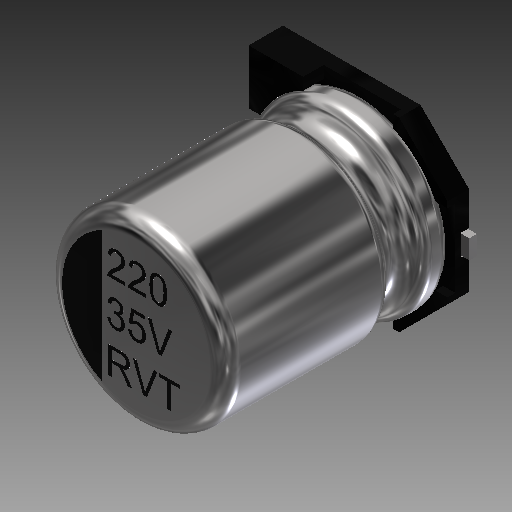
# Autodesk Inventor part: CAPSMD220-35
Saved by Autodesk Inventor 2018 (Build 220112000, 112)
## iProperties
Created: 2017-08-07
Part Number: CAPSMD220-35
Material: Generic
Document SubType Name: Modeling
Designer: joseph.strelchuk
Manufacturer: Standard
Standards Organization: Custom
Density: 1 g/cm^3
Appearance: Semi-Polished
Author: joseph.strelchuk
Autodesk Inventor part; units mm, degrees
ref_plane "YZ Plane" through (0, 0, 0) normal (1, 0, 0) x (0, 1, 0)
ref_plane "XZ Plane" through (0, 0, 0) normal (0, 1, 0) x (-1, 0, 0)
sketch "Sketch11" plane through (0, 0, 0) normal (0, 0, 1) x (1, 0, 0)
  line L0 (-4.15, -4.15) -> (4.15, -4.15)
  line L1 (4.15, -4.15) -> (4.15, 4.15)
  line L2 (4.15, 4.15) -> (-4.15, 4.15)
  line L3 (-4.15, 4.15) -> (-4.15, -4.15)
  line L4 (-4.15, -4.15) -> (4.15, 4.15) construction
  line L5 (4.15, -4.15) -> (-4.15, 4.15) construction
  point P0 (0, 0)
  dimension "d50" = 8.3
  dimension "d51" = 8.3
  constraints: 12 end point, 2 midpoint, 2 parallel, 1 horizontal, 1 perpendicular
  measures "d50" distance of L2.end L1.end
  measures "d51" distance of L1.end L0.end
extrude "Extrusion9" add sketch "Sketch11" along normal blind 1.53
chamfer "Chamfer1" distance 2.16 distance2 2.16 1 edges at (4.15, -4.15, 0.765) measured on face at (-1.3833, -4.15, 0.51)
chamfer "Chamfer2" distance 2.16 distance2 2.16 1 edges at (4.15, 4.15, 0.765) measured on face at (4.15, 0.0567, 0.51)
sketch "Sketch12" plane through (0, 0, 1.53) normal (0, 0, 1) x (1, 0, 0)
  line L0 (4.15, -1.99) -> (1.99, -4.15) construction
  line L1 (1.99, -4.15) -> (-4.15, -4.15) construction
  line L2 (-4.15, -4.15) -> (-4.15, 4.15) construction
  line L3 (-4.15, 4.15) -> (1.99, 4.15) construction
  line L4 (1.99, 4.15) -> (4.15, 1.99) construction
  line L5 (4.15, 1.99) -> (4.15, -1.99) construction
  line L6 (-4.15, 0) -> (4.15, 0) construction
  line L7 (0, 4.15) -> (0, -4.15) construction
  line L8 (-4.15, 1.72) -> (-4.15, -1.72)
  line L9 (-4.15, 4.15) -> (-4.15, -4.15) projected
  line L10 (-1.72, 4.15) -> (1.72, 4.15)
  line L11 (4.15, 1.72) -> (4.15, -1.72)
  line L12 (-1.72, -4.15) -> (1.72, -4.15)
  line L13 (4.15, -1.99) -> (4.15, 1.99) projected
  line L14 (-4.15, -1.72) -> (-3.6113, -1.72)
  line L15 (-4.15, 1.72) -> (-3.6113, 1.72)
  line L16 (-1.72, 4.15) -> (-1.72, 3.6113)
  line L17 (1.72, 4.15) -> (1.72, 3.6113)
  line L18 (4.15, 1.72) -> (3.6113, 1.72)
  line L19 (4.15, -1.72) -> (3.6113, -1.72)
  line L20 (1.72, -4.15) -> (1.72, -3.6113)
  line L21 (-1.72, -4.15) -> (-1.72, -3.6113)
  arc A0 (-3.6113, -1.72) -> (-1.72, -3.6113) centre (0, 0) ccw
  arc A1 (-1.72, 3.6113) -> (-3.6113, 1.72) centre (0, 0) ccw
  arc A2 (1.72, -3.6113) -> (3.6113, -1.72) centre (0, 0) ccw
  arc A3 (3.6113, 1.72) -> (1.72, 3.6113) centre (0, 0) ccw
  dimension "d64" = 3.44
  dimension "d65" = 3.44
  dimension "d66" = 3.44
  dimension "d67" = 3.44
  dimension "d68" = 4
  dimension "d69" = 4
  dimension "d70" = 4
  dimension "d71" = 4
  constraints: 28 end point, 10 midpoint, 8 point on circle, 4 centre point, 4 horizontal, 4 perpendicular, 3 vertical, 2 parallel, 2 point on line, 1 coincident
  measures "d64" distance of L8.start L8.end
  measures "d65" distance of L10.start L10.end
  measures "d66" distance of L11.start L11.end
  measures "d67" distance of L12.start L12.end
  measures "d68" radius of A3
  measures "d69" radius of A1
  measures "d70" radius of A2
  measures "d71" radius of A0
extrude "Extrusion10" cut sketch "Sketch12" against normal blind 0.92
sketch "Sketch13" plane through (0, 0, 1.53) normal (0, 0, 1) x (1, 0, 0)
  line L0 (3.6113, 1.72) -> (4.15, 1.72) projected
  line L1 (4.15, 1.72) -> (4.15, 1.99) projected
  line L2 (1.99, 4.15) -> (4.15, 1.99) projected
  line L3 (1.99, 4.15) -> (1.72, 4.15) projected
  line L4 (1.72, 4.15) -> (1.72, 3.6113) projected
  arc A0 (3.6113, 1.72) -> (1.72, 3.6113) centre (0, 0) ccw projected
  line L5 (4.15, -1.72) -> (3.6113, -1.72) projected
  arc A1 (1.72, -3.6113) -> (3.6113, -1.72) centre (0, 0) ccw projected
  line L6 (1.72, -3.6113) -> (1.72, -4.15) projected
  line L7 (1.72, -4.15) -> (1.99, -4.15) projected
  line L8 (4.15, -1.99) -> (1.99, -4.15) projected
  line L9 (4.15, -1.99) -> (4.15, -1.72) projected
extrude "Extrusion11" cut sketch "Sketch13" against normal blind 0.57
ref_plane "Work Plane1" through (4.15, 0, 0) normal (0, -1, 0) x (0, 0, 1)
sketch "Sketch14" plane through (4.15, 0, 0) normal (0, -1, 0) x (0, 0, 1)
  line L0 (0.61, 2.43) -> (0.61, 5.87) projected
  line L1 (0, 8.3) -> (0, 2.16) projected
  line L2 (0.61, 4.15) -> (10.72, 4.15)
  line L3 (0.61, 4.15) -> (10.7, 4.15)
  line L4 (10.7, 4.15) -> (10.7, 0.85)
  line L5 (0.61, 0.65) -> (0.61, 4.15)
  arc A0 (10, 0.15) -> (10.7, 0.85) centre (10, 0.85) ccw
  line L6 (0.61, 4.15) -> (2.61, 4.15) construction
  line L7 (2.61, 4.15) -> (2.61, 0.15) construction
  arc A1 (3.2974, 0.45) -> (1.9226, 0.45) centre (2.61, 0.15) ccw
  line L8 (10, 0.15) -> (3.7556, 0.15)
  line L9 (1.4644, 0.15) -> (1.11, 0.15)
  arc A2 (3.2974, 0.45) -> (3.7556, 0.15) centre (3.7556, 0.65) ccw
  arc A3 (1.4644, 0.15) -> (1.9226, 0.45) centre (1.4644, 0.65) ccw
  arc A4 (0.61, 0.65) -> (1.11, 0.15) centre (1.11, 0.65) ccw
  point P0 (0, 4.15)
  point P1 (10.7, 0.15)
  point P2 (3.36, 0.15)
  point P3 (1.86, 0.15)
  point P4 (0.63, 2.1134)
  point P5 (0.63, 6.892)
  dimension "d74" = 10.72
  dimension "d75" = 4
  dimension "d76" = 0.7
  dimension "d77" = 2
  dimension "d78" = 1.5
  dimension "d79" = 0.5
  dimension "d80" = 0.3544
  dimension "d81" = 4
  dimension "d82" = 6.2444
  constraints: 16 end point, 12 point on circle, 9 tangent, 5 centre point, 4 point on line, 3 parallel, 3 perpendicular, 2 equal radius, 2 horizontal, 1 coincident, 2 other
  measures "d74" distance from line of L1 L2.end
  measures "d75" distance of L3.end point (10.7, 0.15)
  measures "d76" radius of A0
  measures "d77" distance of L2.start L6.end
  measures "d78" diameter of A1
  measures "d79" radius of A2
  measures "d80" distance of L9.start L9.end
  measures "d81" distance of L6.end L7.end
  measures "d82" distance of L8.start L8.end
revolve "Revolution1" add sketch "Sketch14" angle 360 about axis through (0, 0, 0.61) along (0, 0, 1)
sketch "Sketch15" plane through (0, 0, 0) normal (0, 0, -1) x (-1, 0, 0)
  line L0 (4.5, 0.425) -> (1.12, 0.425) construction
  line L1 (1.12, 0.425) -> (1.12, -0.425) construction
  line L2 (1.12, -0.425) -> (4.5, -0.425) construction
  line L3 (4.5, -0.425) -> (4.5, 0.425) construction
  line L4 (4.15, 4.15) -> (4.15, -4.15) construction
  line L5 (4.15, -4.15) -> (-1.99, -4.15) construction
  line L6 (-1.99, 4.15) -> (4.15, 4.15) construction
  line L7 (1.07, 0.475) -> (4.55, 0.475)
  line L8 (4.55, 0.475) -> (4.55, -0.475)
  line L9 (4.55, -0.475) -> (1.07, -0.475)
  line L10 (1.07, -0.475) -> (1.07, 0.475)
  line L11 (0, -4.15) -> (0, 4.15) construction
  line L12 (-4.15, -1.99) -> (-4.15, 1.99) construction
  line L13 (4.5, -0.425) -> (1.12, 0.425) construction
  line L14 (1.12, -0.425) -> (4.5, 0.425) construction
  line L15 (4.5, 0) -> (-4.5, 0) construction
  line L16 (-4.5, 0.425) -> (-1.12, 0.425) construction
  line L17 (-1.12, 0.425) -> (-1.12, -0.425) construction
  line L18 (-1.12, -0.425) -> (-4.5, -0.425) construction
  line L19 (-4.5, -0.425) -> (-4.5, 0.425) construction
  line L20 (-1.07, 0.475) -> (-4.55, 0.475)
  line L21 (-4.55, 0.475) -> (-4.55, -0.475)
  line L22 (-4.55, -0.475) -> (-1.07, -0.475)
  line L23 (-1.07, -0.475) -> (-1.07, 0.475)
  line L24 (-4.5, -0.425) -> (-1.12, 0.425) construction
  line L25 (-1.12, -0.425) -> (-4.5, 0.425) construction
  point P0 (0, 0)
  dimension "d84" = 3.38
  dimension "d85" = 0.85
  dimension "d91" = 0.05
  dimension "d111" = 9
  dimension "d112" = 8.3
  constraints: 44 end point, 8 symmetric about line, 4 parallel, 3 midpoint, 2 horizontal, 2 perpendicular, 2 point on line, 3 other
  measures "d84" distance of L2.end L1.end
  measures "d85" distance of L1.end L0.end
  measures "d91" distance between parallel lines of L0 L7
  measures "d111" distance of L15.start L15.end
  measures "d112" distance of L11.start L11.end
extrude "Extrusion12" cut sketch "Sketch15" against normal blind 0.34
sketch "Sketch16" plane through (0, 0, 0) normal (0, 0, -1) x (-1, 0, 0)
  line L0 (4.5, 0.425) -> (1.12, 0.425)
  line L1 (1.12, 0.425) -> (1.12, -0.425)
  line L2 (1.12, -0.425) -> (4.5, -0.425)
  line L3 (4.5, -0.425) -> (4.5, 0.425)
  line L4 (0, -4.15) -> (0, 4.15) construction
  line L5 (4.5, -0.425) -> (1.12, 0.425) construction
  line L6 (1.12, -0.425) -> (4.5, 0.425) construction
  line L7 (4.5, 0) -> (-4.5, 0) construction
  line L8 (-1.12, 0.425) -> (-1.12, -0.425)
  line L9 (-4.5, 0.425) -> (-1.12, 0.425)
  line L10 (-1.12, -0.425) -> (-4.5, -0.425)
  line L11 (-4.5, -0.425) -> (-1.12, 0.425) construction
  line L12 (-1.12, -0.425) -> (-4.5, 0.425) construction
  line L13 (-4.5, -0.425) -> (-4.5, 0.425)
  line L14 (4.15, -4.15) -> (-1.99, -4.15) projected
  line L15 (-1.99, 4.15) -> (4.15, 4.15) projected
  line L16 (4.15, 0.475) -> (4.15, -0.475) projected
  line L17 (4.15, 4.15) -> (4.15, 0.475) projected
  line L18 (-4.15, -1.99) -> (-4.15, -0.475) projected
  line L19 (-4.15, -0.475) -> (-4.15, 0.475) projected
  point P0 (0, 0)
  point P1 (0, 0)
  dimension "d113" = 3.38
  dimension "d114" = 0.85
  dimension "d116" = 9
  dimension "d118" = 8.3
  constraints: 28 end point, 4 symmetric about line, 3 midpoint, 2 horizontal, 2 parallel, 1 coincident, 1 perpendicular, 1 point on line
  measures "d113" distance of L2.end L1.end
  measures "d114" distance of L1.end L1.start
  measures "d116" distance of L7.start L7.end
  measures "d118" distance of L4.start L4.end
extrude "Extrusion13" add sketch "Sketch16" against normal blind 0.34
sketch "Sketch17" plane through (0, 0, 10.7) normal (0, 0, 1) x (1, 0, 0)
  circle A0 centre (0, 0) radius 3.3 projected
  line L0 (-3.3, 0) -> (-1.5, 0) construction
  line L1 (-1.5, 2.9394) -> (-1.5, -2.9394)
  point P0 (0, 0)
  dimension "d102" = 1.8
  constraints: 4 end point, 3 point on circle, 1 horizontal, 1 vertical
  measures "d102" distance of L0.start L0.end
extrude "Extrusion14" add sketch "Sketch17" along normal blind 0.001 contours L1 A0 picked at (-1.7221, -0.8298)
sketch "Sketch18" plane through (0, 0, 10.7) normal (0, 0, 1) x (1, 0, 0)
  line L0 (-1.3372, 2.4792) -> (8.132, 2.4792) construction
  line L1 (8.132, 2.4792) -> (8.132, -10.1737) construction
  line L2 (8.132, -10.1737) -> (-1.3372, -10.1737) construction
  line L3 (-1.3372, -10.1737) -> (-1.3372, 2.4792) construction
  line L4 (-1.355, 0.5813) -> (3.616, 0.5813) construction
  line L5 (3.616, 0.5813) -> (3.616, -1.4599) construction
  line L6 (3.616, -1.4599) -> (-1.355, -1.4599) construction
  line L7 (-1.355, -1.4599) -> (-1.355, 0.5813) construction
  line L8 (-1.3639, -1.336) -> (4.226, -1.336) construction
  line L9 (4.226, -1.336) -> (4.226, -3.336) construction
  line L10 (4.226, -3.336) -> (-1.3639, -3.336) construction
  line L11 (-1.3639, -3.336) -> (-1.3639, -1.336) construction
  line L12 (-0.4939, 1.4164) -> (-0.4939, 1.2746)
  line L13 (-0.4939, 1.2746) -> (-1.2869, 1.2746)
  spline S0 degree 2 poles (-1.2869, 1.2746) (-1.2888, 1.3277) (-1.2695, 1.3771) knots 0 0 0 1 1 1
  spline S1 degree 2 poles (-1.2695, 1.3771) (-1.2394, 1.4585) (-1.1058, 1.6149) (-0.9796, 1.7182) knots 0 0 0 1 2 2 2
  spline S2 degree 2 poles (-0.9796, 1.7182) (-0.7848, 1.8792) (-0.6476, 2.0658) (-0.6476, 2.1499) knots 0 0 0 1 2 2 2
  spline S3 degree 2 poles (-0.6476, 2.1499) (-0.6476, 2.2377) (-0.7729, 2.3575) (-0.8735, 2.3575) knots 0 0 0 1 2 2 2
  spline S4 degree 2 poles (-0.8735, 2.3575) (-0.9796, 2.3575) (-1.1067, 2.2295) (-1.1077, 2.117) knots 0 0 0 1 2 2 2
  line L14 (-1.1077, 2.117) -> (-1.2595, 2.1325)
  spline S5 degree 2 poles (-1.2595, 2.1325) (-1.2439, 2.3017) (-1.0409, 2.4792) (-0.8699, 2.4792) knots 0 0 0 1 2 2 2
  spline S6 degree 2 poles (-0.8699, 2.4792) (-0.697, 2.4792) (-0.4958, 2.288) (-0.4958, 2.1463) knots 0 0 0 1 2 2 2
  spline S7 degree 2 poles (-0.4958, 2.1463) (-0.4958, 2.074) (-0.5543, 1.935) (-0.6915, 1.7813) (-0.8497, 1.6469) knots 0 0 0 1 2 3 3 3
  spline S8 degree 2 poles (-0.8497, 1.6469) (-0.9824, 1.5362) (-1.0574, 1.4566) (-1.082, 1.4164) knots 0 0 0 1 2 2 2
  line L15 (-1.082, 1.4164) -> (-0.4939, 1.4164)
  line L16 (0.4381, 1.4164) -> (0.4381, 1.2746)
  line L17 (0.4381, 1.2746) -> (-0.3549, 1.2746)
  spline S9 degree 2 poles (-0.3549, 1.2746) (-0.3567, 1.3277) (-0.3375, 1.3771) knots 0 0 0 1 1 1
  spline S10 degree 2 poles (-0.3375, 1.3771) (-0.3074, 1.4585) (-0.1738, 1.6149) (-0.0476, 1.7182) knots 0 0 0 1 2 2 2
  spline S11 degree 2 poles (-0.0476, 1.7182) (0.1472, 1.8792) (0.2844, 2.0658) (0.2844, 2.1499) knots 0 0 0 1 2 2 2
  spline S12 degree 2 poles (0.2844, 2.1499) (0.2844, 2.2377) (0.1591, 2.3575) (0.0585, 2.3575) knots 0 0 0 1 2 2 2
  spline S13 degree 2 poles (0.0585, 2.3575) (-0.0476, 2.3575) (-0.1747, 2.2295) (-0.1756, 2.117) knots 0 0 0 1 2 2 2
  line L18 (-0.1756, 2.117) -> (-0.3275, 2.1325)
  spline S14 degree 2 poles (-0.3275, 2.1325) (-0.3119, 2.3017) (-0.1089, 2.4792) (0.0622, 2.4792) knots 0 0 0 1 2 2 2
  spline S15 degree 2 poles (0.0622, 2.4792) (0.235, 2.4792) (0.4362, 2.288) (0.4362, 2.1463) knots 0 0 0 1 2 2 2
  spline S16 degree 2 poles (0.4362, 2.1463) (0.4362, 2.074) (0.3777, 1.935) (0.2405, 1.7813) (0.0823, 1.6469) knots 0 0 0 1 2 3 3 3
  spline S17 degree 2 poles (0.0823, 1.6469) (-0.0503, 1.5362) (-0.1253, 1.4566) (-0.15, 1.4164) knots 0 0 0 1 2 2 2
  line L19 (-0.15, 1.4164) -> (0.4381, 1.4164)
  spline S18 degree 2 poles (0.5963, 1.8664) (0.5963, 2.0795) (0.6841, 2.3392) (0.8561, 2.4792) (0.9878, 2.4792) knots 0 0 0 1 2 3 3 3
  spline S19 degree 2 poles (0.9878, 2.4792) (1.0838, 2.4792) (1.2301, 2.4014) (1.3244, 2.2551) (1.3783, 2.0447) (1.3783, 1.8664) knots 0 0 0 1 2 3 4 4 4
  spline S20 degree 2 poles (1.3783, 1.8664) (1.3783, 1.6551) (1.2914, 1.3953) (1.1186, 1.2545) (0.9878, 1.2545) knots 0 0 0 1 2 3 3 3
  spline S21 degree 2 poles (0.9878, 1.2545) (0.814, 1.2545) (0.7152, 1.378) knots 0 0 0 1 1 1
  spline S22 degree 2 poles (0.7152, 1.378) (0.5963, 1.5289) (0.5963, 1.8664) knots 0 0 0 1 1 1
  spline S23 degree 2 poles (0.7481, 1.8664) (0.7481, 1.57) (0.8862, 1.3752) (0.9878, 1.3752) knots 0 0 0 1 2 2 2
  spline S24 degree 2 poles (0.9878, 1.3752) (1.0884, 1.3752) (1.2265, 1.571) (1.2265, 1.8664) knots 0 0 0 1 2 2 2
  spline S25 degree 2 poles (1.2265, 1.8664) (1.2265, 2.1627) (1.0884, 2.3575) (0.9859, 2.3575) knots 0 0 0 1 2 2 2
  spline S26 degree 2 poles (0.9859, 2.3575) (0.8844, 2.3575) (0.824, 2.2716) knots 0 0 0 1 1 1
  spline S27 degree 2 poles (0.824, 2.2716) (0.7481, 2.1618) (0.7481, 1.8664) knots 0 0 0 1 1 1
  line L20 (-1.2846, -0.305) -> (-1.1374, -0.2858)
  spline S28 degree 2 poles (-1.1374, -0.2858) (-1.1118, -0.4111) (-0.9901, -0.5218) (-0.9023, -0.5218) knots 0 0 0 1 2 2 2
  spline S29 degree 2 poles (-0.9023, -0.5218) (-0.798, -0.5218) (-0.6554, -0.3772) (-0.6554, -0.2712) knots 0 0 0 1 2 2 2
  spline S30 degree 2 poles (-0.6554, -0.2712) (-0.6554, -0.1696) (-0.788, -0.0379) (-0.8904, -0.0379) knots 0 0 0 1 2 2 2
  spline S31 degree 2 poles (-0.8904, -0.0379) (-0.9316, -0.0379) (-0.9938, -0.0544) knots 0 0 0 1 1 1
  line L21 (-0.9938, -0.0544) -> (-0.9782, 0.0746)
  spline S32 degree 2 poles (-0.9782, 0.0746) (-0.9627, 0.0728) (-0.9544, 0.0728) knots 0 0 0 1 1 1
  spline S33 degree 2 poles (-0.9544, 0.0728) (-0.8602, 0.0728) (-0.7093, 0.1715) (-0.7093, 0.2731) knots 0 0 0 1 2 2 2
  spline S34 degree 2 poles (-0.7093, 0.2731) (-0.7093, 0.3545) (-0.8191, 0.4606) (-0.906, 0.4606) knots 0 0 0 1 2 2 2
  spline S35 degree 2 poles (-0.906, 0.4606) (-0.9919, 0.4606) (-1.1063, 0.3526) (-1.1227, 0.2438) knots 0 0 0 1 2 2 2
  line L22 (-1.1227, 0.2438) -> (-1.27, 0.2703)
  spline S36 degree 2 poles (-1.27, 0.2703) (-1.2425, 0.4185) (-1.0514, 0.5813) (-0.9087, 0.5813) knots 0 0 0 1 2 2 2
  spline S37 degree 2 poles (-0.9087, 0.5813) (-0.8108, 0.5813) (-0.6453, 0.4971) (-0.5575, 0.3517) (-0.5575, 0.2703) knots 0 0 0 1 2 3 3 3
  spline S38 degree 2 poles (-0.5575, 0.2703) (-0.5575, 0.1926) (-0.6407, 0.0645) (-0.723, 0.027) knots 0 0 0 1 2 2 2
  spline S39 degree 2 poles (-0.723, 0.027) (-0.616, 0.0023) (-0.4989, -0.1522) (-0.4989, -0.2684) knots 0 0 0 1 2 2 2
  spline S40 degree 2 poles (-0.4989, -0.2684) (-0.4989, -0.4248) (-0.7285, -0.6434) (-0.9032, -0.6434) knots 0 0 0 1 2 2 2
  spline S41 degree 2 poles (-0.9032, -0.6434) (-1.0614, -0.6434) (-1.27, -0.455) (-1.2846, -0.305) knots 0 0 0 1 2 2 2
  line L23 (-0.3535, -0.3087) -> (-0.1989, -0.2958)
  spline S42 degree 2 poles (-0.1989, -0.2958) (-0.1816, -0.4093) (-0.0572, -0.5227) (0.0315, -0.5227) knots 0 0 0 1 2 2 2
  spline S43 degree 2 poles (0.0315, -0.5227) (0.1395, -0.5227) (0.2858, -0.3617) (0.2858, -0.2291) knots 0 0 0 1 2 2 2
  spline S44 degree 2 poles (0.2858, -0.2291) (0.2858, -0.1029) (0.145, 0.0435) (0.0297, 0.0435) knots 0 0 0 1 2 2 2
  spline S45 degree 2 poles (0.0297, 0.0435) (-0.0416, 0.0435) (-0.156, -0.0215) (-0.1889, -0.0736) knots 0 0 0 1 2 2 2
  line L24 (-0.1889, -0.0736) -> (-0.327, -0.0553)
  line L25 (-0.327, -0.0553) -> (-0.2108, 0.5612)
  line L26 (-0.2108, 0.5612) -> (0.3855, 0.5612)
  line L27 (0.3855, 0.5612) -> (0.3855, 0.4203)
  line L28 (0.3855, 0.4203) -> (-0.0929, 0.4203)
  line L29 (-0.0929, 0.4203) -> (-0.1578, 0.0984)
  spline S46 degree 2 poles (-0.1578, 0.0984) (-0.0499, 0.1734) (0.069, 0.1734) knots 0 0 0 1 1 1
  spline S47 degree 2 poles (0.069, 0.1734) (0.2264, 0.1734) (0.4422, -0.0443) (0.4422, -0.2154) knots 0 0 0 1 2 2 2
  spline S48 degree 2 poles (0.4422, -0.2154) (0.4422, -0.3791) (0.3471, -0.498) knots 0 0 0 1 1 1
  spline S49 degree 2 poles (0.3471, -0.498) (0.2318, -0.6434) (0.0325, -0.6434) knots 0 0 0 1 1 1
  spline S50 degree 2 poles (0.0325, -0.6434) (-0.1313, -0.6434) (-0.3389, -0.4605) (-0.3535, -0.3087) knots 0 0 0 1 2 2 2
  line L30 (0.98, -0.6233) -> (0.5163, 0.5767)
  line L31 (0.5163, 0.5767) -> (0.6882, 0.5767)
  line L32 (0.6882, 0.5767) -> (1.0001, -0.2949)
  spline S51 degree 2 poles (1.0001, -0.2949) (1.0376, -0.3992) (1.0632, -0.4907) knots 0 0 0 1 1 1
  spline S52 degree 2 poles (1.0632, -0.4907) (1.0907, -0.3928) (1.1273, -0.2949) knots 0 0 0 1 1 1
  line L33 (1.1273, -0.2949) -> (1.452, 0.5767)
  line L34 (1.452, 0.5767) -> (1.6139, 0.5767)
  line L35 (1.6139, 0.5767) -> (1.1437, -0.6233)
  line L36 (1.1437, -0.6233) -> (0.98, -0.6233)
  line L37 (-1.2322, -2.536) -> (-1.2322, -1.336)
  line L38 (-1.2322, -1.336) -> (-0.6999, -1.336)
  spline S53 degree 2 poles (-0.6999, -1.336) (-0.5399, -1.336) (-0.3725, -1.4009) (-0.2728, -1.5646) (-0.2728, -1.6634) knots 0 0 0 1 2 3 3 3
  spline S54 degree 2 poles (-0.2728, -1.6634) (-0.2728, -1.7915) (-0.4383, -1.9662) (-0.6103, -1.99) knots 0 0 0 1 2 2 2
  spline S55 degree 2 poles (-0.6103, -1.99) (-0.5481, -2.0201) (-0.5152, -2.0494) knots 0 0 0 1 1 1
  spline S56 degree 2 poles (-0.5152, -2.0494) (-0.4457, -2.1134) (-0.3835, -2.2095) knots 0 0 0 1 1 1
  line L39 (-0.3835, -2.2095) -> (-0.1758, -2.536)
  line L40 (-0.1758, -2.536) -> (-0.3743, -2.536)
  line L41 (-0.3743, -2.536) -> (-0.5335, -2.2863)
  spline S57 degree 2 poles (-0.5335, -2.2863) (-0.603, -2.1784) (-0.6926, -2.064) (-0.7639, -2.0174) (-0.8005, -2.0082) knots 0 0 0 1 2 3 3 3
  spline S58 degree 2 poles (-0.8005, -2.0082) (-0.828, -2.0028) (-0.8892, -2.0028) knots 0 0 0 1 1 1
  line L42 (-0.8892, -2.0028) -> (-1.0731, -2.0028)
  line L43 (-1.0731, -2.0028) -> (-1.0731, -2.536)
  line L44 (-1.0731, -2.536) -> (-1.2322, -2.536)
  line L45 (-1.0731, -1.8656) -> (-0.7319, -1.8656)
  spline S59 degree 2 poles (-0.7319, -1.8656) (-0.6231, -1.8656) (-0.5005, -1.8207) (-0.4365, -1.7211) (-0.4365, -1.6634) knots 0 0 0 1 2 3 3 3
  spline S60 degree 2 poles (-0.4365, -1.6634) (-0.4365, -1.5784) (-0.56, -1.4686) (-0.6935, -1.4686) knots 0 0 0 1 2 2 2
  line L46 (-0.6935, -1.4686) -> (-1.0731, -1.4686)
  line L47 (-1.0731, -1.4686) -> (-1.0731, -1.8656)
  line L48 (0.3181, -2.536) -> (-0.1457, -1.336)
  line L49 (-0.1457, -1.336) -> (0.0263, -1.336)
  line L50 (0.0263, -1.336) -> (0.3382, -2.2076)
  spline S61 degree 2 poles (0.3382, -2.2076) (0.3757, -2.3119) (0.4013, -2.4034) knots 0 0 0 1 1 1
  spline S62 degree 2 poles (0.4013, -2.4034) (0.4287, -2.3055) (0.4653, -2.2076) knots 0 0 0 1 1 1
  line L51 (0.4653, -2.2076) -> (0.79, -1.336)
  line L52 (0.79, -1.336) -> (0.9519, -1.336)
  line L53 (0.9519, -1.336) -> (0.4818, -2.536)
  line L54 (0.4818, -2.536) -> (0.3181, -2.536)
  line L55 (1.4001, -2.536) -> (1.4001, -1.4778)
  line L56 (1.4001, -1.4778) -> (1.005, -1.4778)
  line L57 (1.005, -1.4778) -> (1.005, -1.336)
  line L58 (1.005, -1.336) -> (1.9562, -1.336)
  line L59 (1.9562, -1.336) -> (1.9562, -1.4778)
  line L60 (1.9562, -1.4778) -> (1.5592, -1.4778)
  line L61 (1.5592, -1.4778) -> (1.5592, -2.536)
  line L62 (1.5592, -2.536) -> (1.4001, -2.536)
  point P0 (0, 0)
  dimension "d15" = 61.595
  constraints: 6 other
emboss "Emboss1" sketch "Sketch18" operation add depth 0.001 direction (0, 0, -1)
equation "\"d69\" = d68"
equation "\"d70\" = d68"
equation "\"d71\" = d68"
equation "\"d75\" = d81"
body "Solid4"
